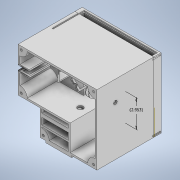
# Autodesk Inventor part: Box
Saved by Autodesk Inventor 2022 (Build 260153000, 153)
## iProperties
Created: 2022-06-14
Part Number: Box
Material: Generic
Document SubType Name: Modeling
Designer: yashm
Density: 1 g/cm^3
Appearance: Default
Author: yashm
Autodesk Inventor part; units mm, degrees
(part 1 of 2)
sketch "Sketch1" plane through (0, 0, 0) normal (0, 0, 1) x (1, 0, 0)
  line L0 (0, 0) -> (145, 0)
  line L1 (145, 0) -> (145, 180)
  line L2 (145, 180) -> (0, 180)
  line L3 (0, 180) -> (0, 0)
  dimension "d0" = 180
  dimension "d1" = 145
  constraints: 8 end point, 2 parallel, 1 horizontal, 1 perpendicular
  measures "d0" distance of L2.end L0.start
  measures "d1" distance of L0.start L0.end
extrude "Extrusion1" add sketch "Sketch1" along normal blind 150
shell "Shell2" thickness 5 outward yes removed faces 1 at (48.3333, 120, 150)
ref_plane "Work Plane1" through (0, 30, 0) normal (0, 1, 0) x (1, 0, 0)
sketch "Sketch4" plane through (0, 30, 0) normal (0, 1, 0) x (1, 0, 0)
  line L0 (53, -95.6365) -> (53, 0)
  line L1 (53, 0) -> (57, 0)
  line L2 (57, 0) -> (57, -95.6365)
  line L3 (0, 0) -> (145, 0) projected
  arc A0 (53, -95.6365) -> (57, -95.6365) centre (55, -100) ccw
  point P0 (55, 0)
  dimension "d8" = 4
  dimension "d10" = 55
  dimension "d12" = 4.8
  dimension "d13" = 100
  constraints: 6 end point, 2 perpendicular, 2 point on circle, 1 centre point, 1 collinear, 1 midpoint, 1 parallel, 1 point on line, 1 vertical
  measures "d8" distance of L0.end L1.end
  measures "d10" distance of L3.start point (55, 0)
  measures "d12" radius of A0
  measures "d13" distance of point (55, 0) A0.centre
extrude "Extrusion2" add sketch "Sketch4" along normal mid plane 4
sketch "Sketch6" plane through (0, 32, 0) normal (0, 1, 0) x (1, 0, 0)
  circle A0 centre (55, -100) radius 2.3
  arc A1 (53, -95.6365) -> (57, -95.6365) centre (55, -100) ccw projected
  point P0 (0, 0)
  dimension "d16" = 4.6
  constraints: 1 centre point, 1 concentric
  measures "d16" diameter of A0
extrude "Extrusion3" cut sketch "Sketch6" against normal blind 4 draft -5
sketch "Sketch8" plane through (0, 30, 0) normal (0, 1, 0) x (1, 0, 0)
  circle A0 centre (55, -100) radius 2.8
  arc A1 (53, -95.6365) -> (57, -95.6365) centre (55, -100) ccw projected
  point P0 (0, 0)
  dimension "d20" = 5.6
  constraints: 1 centre point, 1 concentric
  measures "d20" diameter of A0
extrude "Extrusion4" cut sketch "Sketch8" along normal mid plane 1.3
ref_plane "Work Plane2" through (0, 180, 100) normal (0, 0, 1) x (1, 0, 0)
sketch "Sketch9" plane through (0, 180, 100) normal (0, 0, 1) x (1, 0, 0)
  line L0 (50.2, -152) -> (50.2, -148) projected
  line L1 (59.8, -152) -> (59.8, -148) projected
  line L2 (59.8, -150.6) -> (50.2, -150.6)
  line L3 (50.2, -150.6) -> (50.2, -149.4)
  line L4 (50.2, -149.4) -> (59.8, -149.4)
  line L5 (59.8, -149.4) -> (59.8, -150.6)
  line L6 (59.8, -148) -> (50.2, -148) projected
  point P0 (0, -180)
  point P1 (53, -148)
  point P2 (57, -148)
  point P3 (50.2, -150)
  dimension "d24" = 1.2
  constraints: 8 end point, 3 parallel, 2 midpoint, 1 horizontal, 1 perpendicular
  measures "d24" distance of L2.end L3.end
extrude "Extrusion5" cut sketch "Sketch9" along normal blind 4.8 contours L0 L4 L1 L2
sketch "Sketch10" plane through (0, 180, 100) normal (0, 0, 1) x (1, 0, 0)
  line L0 (52.7, -148) -> (57.3, -148)
  line L1 (57.3, -148) -> (57.3, -152)
  line L2 (57.3, -152) -> (52.7, -152)
  line L3 (52.7, -152) -> (52.7, -148)
  line L4 (52.7, -148) -> (57.3, -148) projected
  line L5 (53, -148) -> (57, -148) projected
  line L6 (53, -148) -> (57, -148) projected
  line L7 (50.2, -152) -> (59.8, -152) projected
  line L8 (52.7, -148) -> (57.3, -148) projected
  line L9 (57, -148) -> (57, -152) projected
  line L10 (57, -148) -> (57, -152) projected
  point P0 (0, -180)
  point P1 (53, -152)
  point P2 (55, -148)
  point P3 (55, -148)
  constraints: 8 end point, 4 midpoint, 2 equal length, 2 parallel, 1 horizontal, 1 perpendicular
extrude "Extrusion6" cut sketch "Sketch10" along normal blind 4.8 contours L0 L9 L2 L3
ref_plane "Work Plane3" through (0, 130, 0) normal (0, 1, 0) x (1, 0, 0)
sketch "Sketch11" plane through (0, 130, 0) normal (0, 1, 0) x (1, 0, 0)
  arc A0 (57, -104.3635) -> (57, -95.6365) centre (55, -100) ccw projected
  line L0 (57, 0) -> (57, -95.6365) projected
  line L1 (53, -95.6365) -> (53, 0) projected
  arc A1 (56.95, -100) -> (53.05, -100) centre (55, -100) ccw projected
  arc A2 (53, -95.6365) -> (52.7, -104.2131) centre (55, -100) ccw projected
  line L2 (52.7, -100) -> (52.7, -104.2131) projected
  line L3 (57, -104.3635) -> (57, -100) projected
  point P0 (0, 0)
sketch "Sketch12" plane through (0, 180, 0) normal (0, 0, 1) x (1, 0, 0)
  line L0 (42.9792, -41.5147) -> (46.5147, -37.9792)
  line L1 (46.5147, -37.9792) -> (67.0208, -58.4853)
  line L2 (67.0208, -58.4853) -> (63.4853, -62.0208)
  line L3 (63.4853, -62.0208) -> (42.9792, -41.5147)
  line L4 (-96, -50) -> (191, -50) projected
  point P0 (0, -180)
  point P1 (55, -50)
  dimension "d30" = 135
  dimension "d31" = 5
  dimension "d32" = 29
  dimension "d33" = 14.5
  dimension "d34" = 2.5
  constraints: 8 end point, 3 perpendicular
  measures "d30" angle of L4 L1
  measures "d31" distance between parallel lines of L1 L3
  measures "d32" distance between parallel lines of L0 L2
  measures "d33" distance from line of point (55, -50) L2
  measures "d34" distance from line of point (55, -50) L3
extrude "Extrusion7" add sketch "Sketch12" along normal blind 115
sketch "Sketch13" plane through (0, 180, 115) normal (0, 0, 1) x (1, 0, 0)
  line L0 (46.5147, -40.8076) -> (64.1924, -58.4853)
  line L1 (64.1924, -58.4853) -> (63.4853, -59.1924)
  line L2 (63.4853, -59.1924) -> (45.8076, -41.5147)
  line L3 (46.5147, -40.8076) -> (45.8076, -41.5147)
  line L4 (63.4853, -62.0208) -> (67.0208, -58.4853) projected
  line L5 (42.9792, -41.5147) -> (63.4853, -62.0208) projected
  line L6 (67.0208, -58.4853) -> (46.5147, -37.9792) projected
  point P0 (0, -180)
  dimension "d41" = 2
  dimension "d42" = 2
  dimension "d43" = 2
  dimension "d44" = 25
  constraints: 8 end point, 2 parallel, 1 perpendicular
  measures "d41" distance between parallel lines of L4 L1
  measures "d42" distance between parallel lines of L5 L2
  measures "d43" distance between parallel lines of L6 L0
  measures "d44" distance between parallel lines of L1 L3
extrude "Extrusion8" cut sketch "Sketch13" against normal blind 27.5
sketch "Sketch14" plane through (63.4853, 117.9792, 115) normal (-0.7071068, -0.7071068, 0) x (-0.7071068, 0.7071068, 0)
  line L0 (95.8173, 120) -> (-38.533, 120) projected
  ellipse E0 centre (14.5, 15) end of major axis (14.5, 10.2) minor radius 3.3941 (16.1263, 10.7869) -> (15.9142, 19.3635) ccw projected
  line L1 (25, 4.5) -> (4, 4.5)
  line L2 (4, 4.5) -> (4, 25.5)
  line L3 (4, 25.5) -> (25, 25.5)
  line L4 (25, 25.5) -> (25, 4.5)
  line L5 (25, 4.5) -> (4, 25.5) construction
  line L6 (4, 4.5) -> (25, 25.5) construction
  point P0 (-38.533, 115)
  dimension "d47" = 21
  dimension "d48" = 21
  constraints: 12 end point, 2 midpoint, 2 parallel, 1 horizontal, 1 perpendicular, 1 other
  measures "d47" distance of L2.end L3.end
  measures "d48" distance of L1.end L2.end
extrude "Extrusion9" cut sketch "Sketch14" against normal blind 5
ref_plane "Work Plane5" through (90, 0, 0) normal (1, 0, 0) x (0, 0, -1)
sketch "Sketch16" plane through (90, 0, 0) normal (1, 0, 0) x (0, 0, -1)
  line L0 (-100, 146.7) -> (0, 146.7)
  line L1 (0, 146.7) -> (0, 113.3)
  line L2 (0, 113.3) -> (-100, 113.3)
  line L3 (-150, 180) -> (-150, 0) projected
  line L4 (0, 121.5147) -> (0, 117.9792) projected
  line L5 (0, 117.9792) -> (0, 138.4853) projected
  line L6 (0, 138.4853) -> (0, 142.0208) projected
  line L7 (0, 142.0208) -> (0, 121.5147) projected
  line L8 (0, 28) -> (0, 32) projected
  line L9 (0, 32) -> (0, 28) projected
  line L10 (0, 0) -> (0, 180) projected
  line L11 (0, 180) -> (0, 0) projected
  arc A0 (-100, 146.7) -> (-100, 113.3) centre (-100, 130) ccw
  point P0 (-100, 130)
  dimension "d370" = 33.4
  dimension "d371" = 0
  dimension "d372" = 16.7
  dimension "d373" = 100
  dimension "d374" = 130
  constraints: 6 end point, 2 point on circle, 1 centre point, 1 point on line
  measures "d370" distance between parallel lines of L2 L0
  measures "d371" horizontal distance of L0.start A0.centre
  measures "d372" radius of A0
  measures "d373" distance from line of L7 A0.centre
  measures "d374" vertical distance of point (0, 0) A0.centre
extrude "Extrusion10" add sketch "Sketch16" along normal mid plane 10
sketch "Sketch17" plane through (95, 0, 0) normal (1, 0, 0) x (0, 0, -1)
  circle A0 centre (-100, 130) radius 10
  arc A1 (-100, 146.7) -> (-100, 113.3) centre (-100, 130) ccw projected
  point P0 (0, 0)
  dimension "d57" = 20
  constraints: 1 centre point, 1 concentric
  measures "d57" diameter of A0
extrude "Extrusion11" cut sketch "Sketch17" against normal blind 14
ref_plane "Work Plane6" through (115, 0, 0) normal (1, 0, 0) x (0, 0, -1)
ref_plane "Work Plane7" through (5, 0, 0) normal (1, 0, 0) x (0, 0, -1)
ref_plane "Work Plane8" through (0, 180, 100) normal (0, 0, 1) x (1, 0, 0)
ref_plane "Work Plane9" through (1460.5, 0, 0) normal (1, 0, 0) x (0, 0, -1)
ref_plane "Work Plane10" through (57.5, 0, 0) normal (1, 0, 0) x (0, 0, -1)
sketch "Sketch27" plane through (0, 0, -5) normal (0, 0, -1) x (-1, 0, 0)
  line L0 (65, 185) -> (5, 185)
  line L1 (5, 185) -> (5, 65)
  line L2 (5, 65) -> (65, 65)
  line L3 (65, 65) -> (65, 185)
  line L4 (5, 185) -> (5, -5) projected
  point P0 (0, 0)
  dimension "d92" = 120
  dimension "d93" = 60
  constraints: 8 end point, 2 parallel, 2 point on line, 1 horizontal, 1 perpendicular
  measures "d92" distance of L0.end L1.end
  measures "d93" distance between parallel lines of L3 L1
extrude "Extrusion18" add sketch "Sketch27" against normal blind 155
sketch "Sketch28" plane through (0, 0, 150) normal (0, 0, 1) x (1, 0, 0)
  line L0 (-60, 180) -> (-5, 180)
  line L1 (-5, 180) -> (-5, 70)
  line L2 (-5, 70) -> (-60, 70)
  line L3 (-60, 70) -> (-60, 180)
  line L4 (-5, 65) -> (-5, -5) projected
  line L5 (-65, 65) -> (-5, 65) projected
  line L6 (-65, 185) -> (-65, 65) projected
  line L7 (150, 185) -> (-65, 185) projected
  point P0 (0, 0)
  point P1 (-5, 185)
  dimension "d96" = 0
  dimension "d97" = 5
  dimension "d98" = 5
  dimension "d99" = 5
  constraints: 8 end point, 2 parallel, 1 horizontal, 1 perpendicular
  measures "d96" distance from line of L4 L1.end
  measures "d97" distance between parallel lines of L5 L2
  measures "d98" distance between parallel lines of L6 L3
  measures "d99" distance between parallel lines of L7 L0
extrude "Extrusion19" cut sketch "Sketch28" against normal blind 200
sketch "Sketch45" plane through (0, 0, -5) normal (0, 0, -1) x (-1, 0, 0)
  line L0 (5, 180) -> (60, 180)
  line L1 (60, 180) -> (60, 70)
  line L2 (60, 70) -> (5, 70)
  line L3 (5, 70) -> (5, 180)
  point P0 (0, 0)
  constraints: 8 end point, 3 coincident, 2 parallel, 1 horizontal, 1 perpendicular
extrude "Extrusion29" add sketch "Sketch45" against normal blind 5
sketch "Sketch57" plane through (0, 0, 150) normal (0, 0, 1) x (1, 0, 0)
  line L0 (145, 180) -> (0, 180) projected
  line L1 (-5, 70) -> (-60, 70) projected
  line L2 (0, 180) -> (-5, 180)
  line L3 (-5, 180) -> (-5, 70)
  line L4 (-5, 70) -> (0, 70)
  line L5 (0, 70) -> (0, 180)
  point P0 (0, 0)
  constraints: 8 end point, 2 parallel, 1 horizontal, 1 perpendicular
extrude "Extrusion36" cut sketch "Sketch57" against normal blind 150
ref_plane "Work Plane12" through (115, 0, 150) normal (1, 0, 0) x (0, 0, -1)
sketch "Sketch64" plane through (-60, 70, 150) normal (1, 0, 0) x (0, 0, -1)
  line L0 (62, 66) -> (0, 66)
  line L1 (0, 66) -> (0, 70)
  line L2 (0, 70) -> (66, 70)
  line L3 (66, 70) -> (66, 50)
  line L4 (66, 50) -> (0, 50)
  line L5 (0, 50) -> (0, 54)
  line L6 (0, 54) -> (62, 54)
  line L7 (62, 54) -> (62, 66)
  circle A0 centre (50, 60) radius 10 projected
  line L8 (0, 0) -> (0, 110) projected
  point P0 (150, -70)
  point P1 (0, 68)
  dimension "d219" = 4
  dimension "d220" = 4
  dimension "d221" = 12
  dimension "d223" = 6
  dimension "d224" = 12
  constraints: 16 end point, 6 perpendicular, 2 equal length, 1 horizontal, 1 midpoint, 1 parallel, 1 point on line
  measures "d219" distance of L0.end L1.end
  measures "d220" distance between parallel lines of L3 L7
  measures "d221" distance of L6.end L0.start
  measures "d223" distance from line of L0 A0.centre
  measures "d224" distance from line of A0.centre L7
extrude "Extrusion43" add sketch "Sketch64" along normal blind 25 contours L0 A0 L2 L3 L4 L6 L7 | L0 A0 | L0 L1 L2 A0 | A0 L6 | A0 L4 L5 L6
sketch "Sketch67" plane through (-65, 65, -5) normal (-1, 0, 0) x (0, 0, 1)
  line L0 (89, 75) -> (155, 75) projected
  line L1 (89, 55) -> (89, 75) projected
  line L2 (155, 55) -> (89, 55) projected
  line L3 (89, 55) -> (155, 55) projected
  line L4 (89, 55) -> (89, 75)
  line L5 (155, 75) -> (89, 75) projected
  line L6 (89, 75) -> (155, 75)
  line L7 (155, 75) -> (155, 55)
  line L8 (155, 55) -> (89, 55)
  line L9 (155, 120) -> (155, 0) projected
  point P0 (5, -65)
  point P1 (155, 65)
  point P2 (118, 75)
  constraints: 8 end point, 2 perpendicular, 2 point on line, 1 collinear, 1 midpoint
extrude "Extrusion44" cut sketch "Sketch67" against normal blind 3
sketch "Sketch68" plane through (-62, 65, -5) normal (-1, 0, 0) x (0, 0, 1)
  line L0 (155, 71) -> (93, 71) projected
  line L1 (93, 71) -> (93, 59) projected
  line L2 (89, 55) -> (89, 75) projected
  line L3 (89, 75) -> (155, 75) projected
  line L4 (93, 59) -> (155, 59) projected
  line L5 (155, 55) -> (89, 55) projected
  line L6 (91, 73) -> (91, 57)
  line L7 (91, 57) -> (155, 57)
  line L8 (155, 57) -> (155, 73)
  line L9 (155, 73) -> (91, 73)
  line L10 (155, 75) -> (155, 55) projected
  point P0 (5, -65)
  dimension "d229" = 2
  dimension "d230" = 2
  dimension "d231" = 2
  dimension "d232" = 0
  constraints: 8 end point, 3 perpendicular, 1 vertical
  measures "d229" distance between parallel lines of L9 L0
  measures "d230" distance between parallel lines of L6 L1
  measures "d231" distance between parallel lines of L7 L4
  measures "d232" distance between parallel lines of L8 L10
extrude "Extrusion45" cut sketch "Sketch68" against normal blind 2 contours L8 L4 L1 L0 | L0 L1 L4 L8 L7 L6 L9
ref_plane "Work Plane13" through (0, 0, 65) normal (0, 0, 1) x (1, 0, 0)
sketch "Sketch71" plane through (0, 0, 65) normal (0, 0, 1) x (1, 0, 0)
  line L0 (145, 180) -> (-60, 180) projected
  line L1 (-60, 180) -> (30, 180)
  line L2 (30, 180) -> (30, 70)
  line L3 (30, 70) -> (-60, 70)
  line L4 (-60, 70) -> (-60, 180)
  line L5 (0, 70) -> (-60, 70) projected
  point P0 (0, 0)
  point P1 (30, 180)
  dimension "d236" = 90
  constraints: 8 end point, 2 parallel, 1 horizontal, 1 perpendicular, 1 point on line
  measures "d236" distance between parallel lines of L4 L2
extrude "Extrusion46" add sketch "Sketch71" along normal mid plane 4
sketch "Sketch74" plane through (0, 0, 67) normal (0, 0, 1) x (1, 0, 0)
  line L0 (0, 70) -> (30, 70) projected
  line L1 (0, 70) -> (30, 70)
  line L2 (30, 70) -> (30, 180) projected
  line L3 (30, 70) -> (30, 180)
  line L4 (30, 180) -> (27, 180)
  line L5 (-60, 180) -> (30, 180) projected
  line L6 (30, 180) -> (27, 180)
  line L7 (27, 180) -> (27, 73)
  line L8 (27, 73) -> (0, 73)
  line L9 (0, 73) -> (0, 70)
  point P0 (0, 0)
  dimension "d239" = 3
  dimension "d240" = 3
  constraints: 14 end point, 3 collinear, 2 perpendicular, 1 point on line, 1 vertical
  measures "d239" distance between parallel lines of L8 L0
  measures "d240" distance between parallel lines of L2 L7
extrude "Extrusion47" add sketch "Sketch74" against normal through all
sketch "Sketch76" plane through (-65, 65, -5) normal (-1, 0, 0) x (0, 0, 1)
  line L0 (68.001, 120) -> (68.001, 0)
  line L1 (68, 115) -> (68, 5) projected
  line L2 (155, 0) -> (0, 0) projected
  line L3 (68.001, 0) -> (0, 0)
  line L4 (0, 0) -> (0, 120) projected
  line L5 (0, 0) -> (0, 120)
  line L6 (0, 120) -> (68.001, 120)
  line L7 (0, 120) -> (155, 120) projected
  point P0 (5, -65)
  point P1 (68.001, 0)
  constraints: 6 end point, 3 collinear, 1 vertical, 3 other
extrude "Extrusion48" cut sketch "Sketch76" against normal blind 5
ref_plane "Work Plane14" through (-25, 70, 150) normal (1, 0, 0) x (0, 0, -1)
sketch "Sketch85" plane through (0, 0, 67) normal (0, 0, 1) x (1, 0, 0)
  line L0 (-32.5, 136) -> (-20.5, 136)
  line L1 (-20.5, 136) -> (-20.5, 124)
  line L2 (-20.5, 124) -> (-32.5, 124)
  line L3 (-32.5, 124) -> (-32.5, 136)
  line L4 (-60, 124) -> (-35, 124) projected
  line L5 (-60, 136) -> (-35, 136) projected
  line L6 (-60, 124) -> (-60, 136) projected
  line L7 (-35, 136) -> (-35, 124) projected
  point P0 (0, 0)
  dimension "d275" = 12
  dimension "d571" = 12
  dimension "d572" = 25
  dimension "d575" = 0
  constraints: 8 end point, 2 parallel, 2 perpendicular, 1 horizontal
  measures "d275" distance of L0.start L0.end
  measures "d571" distance between parallel lines of L4 L5
  measures "d572" distance between parallel lines of L6 L7
  measures "d575" distance between parallel lines of L5 L0
extrude "sample lens stand" add sketch "Sketch85" along normal blind 19.74 contours L0 L1 L2 L3
ref_plane "Work Plane15" through (0, 0, 77) normal (0, 0, 1) x (1, 0, 0)
ref_plane "Work Plane21" through (0, 0, 79) normal (0, 0, 1) x (1, 0, 0)
sketch "Sketch89" plane through (0, 0, 67) normal (0, 0, 1) x (1, 0, 0)
  line L0 (-12.14, 140) -> (-8.14, 140)
  line L1 (-8.14, 140) -> (-8.14, 144)
  line L2 (-8.14, 144) -> (-12.14, 144)
  line L3 (-12.14, 144) -> (-12.14, 140)
  circle A0 centre (-5.14, 130) radius 5 projected
  line L4 (-35, 140) -> (-35, 136) projected
  point P0 (0, 0)
  dimension "d285" = 4
  dimension "d286" = 4
  dimension "d287" = 10
  dimension "d309" = 3
  dimension "d682" = 22.86
  constraints: 8 end point, 2 parallel, 1 horizontal, 1 perpendicular
  measures "d285" distance of L2.end L0.start
  measures "d286" distance of L1.end L2.end
  measures "d287" distance from line of L0 A0.centre
  measures "d309" distance from line of A0.centre L1
  measures "d682" distance between parallel lines of L4 L3
extrude "Extrusion57" add sketch "Sketch89" along normal blind 35 contours L3 L2 L1 L0
sketch "Sketch90" plane through (-12.14, 140, 67) normal (0, -1, 0) x (1, 0, 0)
  line L0 (-2.7175, 26.1109) -> (14.9602, 43.7886)
  line L1 (14.9602, 43.7886) -> (17.7886, 40.9602)
  line L2 (17.7886, 40.9602) -> (0.1109, 23.2825)
  line L3 (0.1109, 23.2825) -> (-2.7175, 26.1109)
  line L4 (0, 0) -> (0, 35) projected
  line L5 (0, 35) -> (4, 35) projected
  point P0 (12.14, -67)
  point P1 (4, 30)
  dimension "d291" = 45
  dimension "d292" = 5
  dimension "d293" = 4
  dimension "d294" = 25
  dimension "d295" = 2
  dimension "d296" = 7.5
  dimension "d297" = 4
  constraints: 8 end point, 3 perpendicular
  measures "d291" angle of L4 L0
  measures "d292" distance from line of point (4, 30) L5
  measures "d293" distance between parallel lines of L2 L0
  measures "d294" distance between parallel lines of L1 L3
  measures "d295" distance from line of L2 point (4, 30)
  measures "d296" distance from line of L3 point (4, 30)
  measures "d297" distance from line of L4 point (4, 30)
extrude "Extrusion58" add sketch "Sketch90" along normal blind 30 and the other way blind 30
sketch "Sketch91" plane through (-14.8575, 110, 93.1109) normal (-0.7071068, 0, 0.7071068) x (0.7071068, 0, 0.7071068)
  line L0 (3, 60) -> (22, 60)
  line L1 (22, 60) -> (22, 3)
  line L2 (22, 3) -> (3, 3)
  line L3 (3, 3) -> (3, 60)
  line L4 (0, 60) -> (25, 60) projected
  line L5 (25, 0) -> (0, 0) projected
  line L6 (25, 60) -> (25, 0) projected
  line L7 (0, 60) -> (0, 0) projected
  point P0 (-55.3335, -110)
  dimension "d302" = 3
  dimension "d303" = 3
  dimension "d304" = 3
  constraints: 8 end point, 2 parallel, 1 horizontal, 1 perpendicular, 1 point on line
  measures "d302" distance between parallel lines of L5 L2
  measures "d303" distance between parallel lines of L6 L1
  measures "d304" distance between parallel lines of L7 L3
extrude "Extrusion59" cut sketch "Sketch91" along normal blind 5 and the other way blind 10 contours L0 L1 L2 L3
sketch "Sketch94" plane through (-12.14, 170, 67) normal (0, 1, 0) x (1, 0, 0)
  line L0 (14.9602, -41.6673) -> (-0.5962, -26.1109)
  line L1 (-0.5962, -26.1109) -> (0.1109, -25.4038)
  line L2 (0.1109, -25.4038) -> (15.6673, -40.9602)
  line L3 (15.6673, -40.9602) -> (14.9602, -41.6673)
  line L4 (-2.7175, -26.1109) -> (-0.5962, -28.2322) projected
  line L5 (0.1109, -23.2825) -> (-2.7175, -26.1109) projected
  line L6 (14.9602, -43.7886) -> (17.7886, -40.9602) projected
  line L7 (2.2322, -25.4038) -> (0.1109, -23.2825) projected
  line L8 (12.8388, -41.6673) -> (14.9602, -43.7886) projected
  point P0 (12.14, 67)
  dimension "d310" = 25
  dimension "d311" = 4
  dimension "d312" = 1.5
  dimension "d313" = 1.5
  dimension "d314" = 1.5
  dimension "d315" = 1.5
  constraints: 8 end point, 4 parallel
  measures "d310" distance between parallel lines of L6 L5
  measures "d311" distance between parallel lines of L7 L4
  measures "d312" distance between parallel lines of L5 L1
  measures "d313" distance between parallel lines of L6 L3
  measures "d314" distance between parallel lines of L8 L0
  measures "d315" distance between parallel lines of L7 L2
extrude "Extrusion60" cut sketch "Sketch94" against normal blind 42
sketch "Sketch98" plane through (0, 0, 0) normal (0, 0, 1) x (1, 0, 0)
  line L0 (0, 65) -> (0, 70)
  line L1 (0, 70) -> (77, 70)
  line L2 (77, 70) -> (77, 0)
  line L3 (77, 0) -> (72, 0)
  line L4 (72, 0) -> (72, 65)
  line L5 (72, 65) -> (0, 65)
  line L6 (-65, 65) -> (-5, 65) projected
  line L7 (0, 70) -> (-60, 70) projected
  line L8 (145, 0) -> (0, 0) projected
  line L9 (57, 32) -> (57, 28) projected
  point P0 (74.5, 0)
  dimension "d328" = 5
  dimension "d329" = 5
  dimension "d330" = 15
  constraints: 12 end point, 6 perpendicular, 1 midpoint, 1 point on line, 1 vertical
  measures "d328" distance of L2.end L3.end
  measures "d329" distance between parallel lines of L6 L7
  measures "d330" distance between parallel lines of L9 L4
extrude "Extrusion64" add sketch "Sketch98" along normal blind 150
sketch "Sketch99" plane through (-60, 70, 67) normal (0, 1, 0) x (1, 0, 0)
  circle A0 centre (115, -33) radius 7.5
  arc A1 (117, -37.3635) -> (117, -28.6365) centre (115, -33) ccw projected
  point P0 (60, 67)
  dimension "d333" = 15
  constraints: 1 centre point, 1 concentric
  measures "d333" diameter of A0
extrude "Extrusion65" cut sketch "Sketch99" against normal blind 5
ref_plane "Work Plane16" through (0, 0, -20) normal (0, 0, -1) x (-1, 0, 0)
sketch "Sketch111" plane through (63.4853, 117.9792, 115) normal (-0.7071068, -0.7071068, 0) x (-0.7071068, 0.7071068, 0)
  line L0 (0, 115) -> (0, 0) projected
  line L1 (29, 115) -> (29, 0) projected
  arc A0 (18.5, 0) -> (10.5, 0) centre (14.5, 0) ccw
  line L2 (29, 0) -> (0, 0) projected
  line L3 (18.5, 0) -> (10.5, 0)
  line L4 (4, 4.5) -> (25, 4.5) projected
  point P0 (-38.533, 115)
  dimension "d382" = 29
  dimension "d383" = 14.5
  dimension "d384" = 4
  constraints: 2 end point, 2 point on circle, 1 centre point, 1 midpoint, 1 parallel, 1 point on line
  measures "d382" distance between parallel lines of L0 L1
  measures "d383" distance from line of L1 A0.centre
  measures "d384" radius of A0
extrude "Extrusion69" cut sketch "Sketch111" against normal blind 5
sketch "Sketch112" plane through (150, -5, -5) normal (1, 0, 0) x (0, 0, -1)
  circle A0 centre (-105, 135) radius 10 projected
  circle A1 centre (-105, 135) radius 5
  point P0 (-5, 5)
  dimension "d387" = 10
  constraints: 1 centre point, 1 coincident
  measures "d387" diameter of A1
extrude "Extrusion70" cut sketch "Sketch112" against normal blind 5 contours A1
sketch "Sketch114" plane through (0, 0, -5) normal (0, 0, -1) x (-1, 0, 0)
  line L0 (5, -5) -> (-150, -5) projected
  line L1 (5, -5) -> (-150, -5)
  line L2 (-150, -5) -> (-150, 185) projected
  line L3 (-150, -5) -> (-150, 185)
  line L4 (-150, 185) -> (60, 185) projected
  line L5 (-150, 185) -> (60, 185)
  line L6 (5, 65) -> (60, 65) projected
  line L7 (60, 185) -> (60, 65)
  line L8 (5, 65) -> (5, -5) projected
  line L9 (60, 65) -> (5, 65)
  line L10 (5, 65) -> (5, -5)
  point P0 (0, 0)
  constraints: 12 end point, 3 collinear, 2 perpendicular, 1 horizontal
extrude "Extrusion71" add sketch "Sketch114" along normal blind 20
sketch "Sketch115" plane through (-5, -5, 150) normal (0, -1, 0) x (1, 0, 0)
  line L0 (150, -170) -> (5, -170)
  line L1 (5, -170) -> (5, -155)
  line L2 (5, -155) -> (150, -155)
  line L3 (150, -155) -> (150, -170)
  line L4 (155, -175) -> (0, -175) projected
  line L5 (155, 0) -> (155, -175) projected
  line L6 (0, -175) -> (0, 0) projected
  point P0 (5, -150)
  dimension "d393" = 5
  dimension "d394" = 5
  dimension "d395" = 5
  dimension "d396" = 15
  constraints: 8 end point, 2 parallel, 1 horizontal, 1 perpendicular
  measures "d393" distance between parallel lines of L0 L4
  measures "d394" distance between parallel lines of L3 L5
  measures "d395" distance between parallel lines of L6 L1
  measures "d396" distance between parallel lines of L0 L2
extrude "Extrusion72" cut sketch "Sketch115" against normal blind 67
sketch "Sketch117" plane through (-65, 185, 150) normal (0, 1, 0) x (1, 0, 0)
  line L0 (10, 170) -> (210, 170)
  line L1 (210, 170) -> (210, 155)
  line L2 (210, 155) -> (10, 155)
  line L3 (10, 155) -> (10, 170)
  line L4 (5, 86.999) -> (5, 175) projected
  line L5 (215, 175) -> (215, 0) projected
  line L6 (5, 175) -> (215, 175) projected
  point P0 (65, 150)
  dimension "d401" = 15
  dimension "d402" = 5
  dimension "d403" = 5
  dimension "d404" = 5
  constraints: 8 end point, 2 parallel, 1 horizontal, 1 perpendicular
  measures "d401" distance of L0.end L1.end
  measures "d402" distance between parallel lines of L4 L3
  measures "d403" distance between parallel lines of L5 L1
  measures "d404" distance between parallel lines of L0 L6
extrude "Extrusion73" cut sketch "Sketch117" against normal blind 117
sketch "Sketch124" plane through (-5, -5, 150) normal (0, -1, 0) x (1, 0, 0)
  arc A0 (57.8181, -50) -> (62, -49.1279) centre (60, -50) ccw projected
  circle A1 centre (60, -50) radius 5
  point P0 (5, -150)
  constraints: 1 centre point, 1 coincident
extrude "Extrusion78" cut sketch "Sketch124" against normal blind 10
sketch "Sketch125" plane through (0, 0, 150) normal (0, 1, 0) x (1, 0, 0)
  circle A0 centre (55, 50) radius 5 projected
  circle A1 centre (55, 50) radius 5
  point P0 (0, 150)
  constraints: 1 centre point, 1 coincident
extrude "Extrusion79" add sketch "Sketch125" along normal mid plane 2.6
sketch "Sketch126" plane through (55, 1.3, 100) normal (0, 1, 0) x (1, 0, 0)
  circle A0 centre (0, 0) radius 1.775
  point P0 (-55, 100)
  dimension "d423" = 3.55
  constraints: 1 centre point
  measures "d423" diameter of A0
extrude "Extrusion80" cut sketch "Sketch126" against normal blind 2.6
sketch "Sketch127" plane through (55, -1.3, 100) normal (0, -1, 0) x (1, 0, 0)
  circle A0 centre (0, 0) radius 2.8
  point P0 (-55, -100)
  dimension "d426" = 5.6
  constraints: 1 centre point
  measures "d426" diameter of A0
extrude "Extrusion81" cut sketch "Sketch127" against normal blind 1.2
sketch "Sketch128" plane through (55, -0.1, 100) normal (0, -1, 0) x (1, 0, 0)
  circle A0 centre (0, 0) radius 2.1
  point P0 (-55, -100)
  dimension "d429" = 4.2
  constraints: 1 centre point
  measures "d429" diameter of A0
extrude "Extrusion82" cut sketch "Sketch128" against normal blind 0.1
sketch "Sketch131" plane through (0, 0, 67) normal (0, 0, 1) x (1, 0, 0)
  line L0 (-9.9078, 170) -> (-9.9078, 144) projected
  line L1 (-14.8575, 170) -> (-12.7362, 170) projected
  line L2 (5.6486, 170) -> (5.6486, 110) construction
  line L3 (2.8202, 110) -> (-14.8575, 110) projected
  line L4 (5.6486, 110) -> (2.8202, 110) projected
  line L5 (-14.8575, 110) -> (5.6486, 110)
  line L6 (0.6988, 170) -> (5.6486, 170)
  line L7 (5.6486, 161.5372) -> (5.6486, 170)
  line L8 (-60, 70) -> (-60, 180) projected
  line L9 (-14.8575, 170) -> (-9.9078, 170)
  line L10 (-9.9078, 113) -> (0.6988, 113)
  line L11 (-14.8575, 170) -> (-14.8575, 110) projected
  line L12 (-9.9078, 170) -> (-9.9078, 144)
  line L13 (-60, 65) -> (-60, 185) projected
  line L14 (-9.9078, 144) -> (-14.8575, 144)
  line L15 (-14.8575, 170) -> (-14.8575, 144)
  line L16 (-14.8575, 110) -> (-14.8575, 113)
  line L17 (0.6988, 113) -> (-14.8575, 113)
  line L18 (-35, 124) -> (-35, 120) projected
  line L19 (0.6988, 170) -> (0.6988, 140)
  line L20 (0.6988, 140) -> (5.6486, 140)
  line L21 (5.6486, 161.5372) -> (5.6486, 140)
  line L22 (0.6988, 113) -> (5.6486, 113)
  line L23 (5.6486, 110) -> (5.6486, 113)
  point P0 (0, 0)
  constraints: 30 end point, 5 perpendicular, 5 point on line, 2 collinear, 1 horizontal, 1 midpoint, 1 parallel, 1 vertical
extrude "Extrusion85" add sketch "Sketch131" along normal up to surface surface through (-12.0291, 140, 90.2825) normal (0.7071068, 0, -0.7071068)
sketch "Sketch132" plane through (-12.14, 170, 67) normal (0, 1, 0) x (1, 0, 0)
  line L0 (14.6066, -39.8995) -> (15.6673, -40.9602) projected
  line L1 (14.6066, -39.8995) -> (14.3102, -37.4818)
  line L2 (15.6673, -38.8388) -> (12.8388, -36.0104) projected
  line L3 (15.6673, -38.8388) -> (14.6066, -39.8995) projected
  line L4 (15.6673, -38.8388) -> (14.6066, -39.8995)
  line L5 (14.3102, -37.4818) -> (15.6673, -38.8388)
  line L6 (-2.7175, -26.1109) -> (-2.7175, -20.4541)
  line L7 (-2.7175, -20.4541) -> (0.1109, -23.2825)
  line L8 (0.1109, -23.2825) -> (-2.7175, -20.4541) projected
  line L9 (0.1109, -23.2825) -> (-2.7175, -26.1109) projected
  line L10 (-2.7175, -26.1109) -> (0.1109, -23.2825)
  point P0 (12.14, 67)
  constraints: 13 end point, 3 collinear, 1 point on line, 1 vertical
extrude "Extrusion86" add sketch "Sketch132" against normal blind 44
sketch "Sketch134" plane through (145, 0, 0) normal (0, 0, 1) x (1, 0, 0)
  line L0 (-68, 70) -> (-205, 70) projected
  line L1 (-150, -5) -> (5, -5) projected
  point P0 (-145, 0)
  dimension "d444" = 75
  measures "d444" distance between parallel lines of L0 L1
sketch "Sketch135" plane through (0, 0, 150) normal (0, 0, 1) x (1, 0, 0)
  line L0 (-60, 160) -> (-60, 179.9274)
  line L1 (-60, 185) -> (-60, 65) projected
  line L2 (27, 180) -> (-60, 180) projected
  line L3 (-60, 180) -> (-40, 180)
  arc A0 (-60, 160) -> (-40, 180) centre (-60, 180) ccw
  line L4 (145, 160) -> (145, 180)
  line L5 (145, 180) -> (125, 180)
  line L6 (145, 20) -> (145, 0)
  line L7 (145, 0) -> (125, 0)
  line L8 (20, 0) -> (0, 0)
  line L9 (0, 0) -> (0, 20)
  line L10 (0, -5) -> (0, 62) projected
  line L11 (-40, 70) -> (-60, 70)
  line L12 (-60, 70) -> (-60, 90)
  arc A1 (125, 180) -> (145, 160) centre (145, 180) ccw
  arc A2 (145, 20) -> (125, 0) centre (145, 0) ccw
  arc A3 (20, 0) -> (0, 20) centre (0, 0) ccw
  arc A4 (-40, 70) -> (-60, 90) centre (-60, 70) ccw
  dimension "d446" = 20
  constraints: 22 end point, 10 point on circle, 7 coincident, 5 centre point, 4 equal radius, 3 perpendicular, 2 horizontal, 2 point on line, 2 vertical, 1 collinear
  measures "d446" distance of L4.start L4.end
extrude "Extrusion87" add sketch "Sketch135" against normal up to next
sketch "Sketch137" plane through (-12.7362, 128, 93.1109) normal (0.7071068, 0, 0.7071068) x (0.7071068, 0, -0.7071068)
  line L0 (1, 0) -> (0, 0)
  line L1 (0, 0) -> (0, 42) projected
  line L2 (1, 0) -> (0, 0)
  line L3 (0, 0) -> (0, 25)
  line L4 (0, 25) -> (1, 25)
  line L5 (1, 25) -> (1, 0)
  point P0 (74.8452, -128)
  point P1 (0, 1)
  dimension "d449" = 25
  constraints: 10 end point, 2 parallel, 1 horizontal, 1 perpendicular, 1 point on line
  measures "d449" distance of L4.end L0.start
sketch "Sketch138" plane through (2.8202, 110, 110.7886) normal (-0.7071068, 0, 0.7071068) x (0.7071068, 0, 0.7071068)
  line L0 (-23.5, 60) -> (-23.5, 18) projected
  line L1 (-1.5, 60) -> (-1.5, 18) projected
  line L2 (-23.5, 60) -> (-1.5, 60)
  line L3 (-1.5, 60) -> (-1.5, 41.5)
  line L4 (-1.5, 41.5) -> (-23.5, 41.5)
  line L5 (-23.5, 41.5) -> (-23.5, 60)
  point P0 (-80.3335, -110)
  point P1 (-23.5, 43)
  point P2 (-23.5, 43)
  point P3 (-23.5, 43)
  dimension "d450" = 1.5
  constraints: 8 end point, 2 parallel, 1 horizontal, 1 perpendicular, 1 point on line
  measures "d450" distance from line of L4 point (-23.5, 43)
extrude "Extrusion88" add sketch "Sketch138" against normal blind 4
extrude "Extrusion89" cut sketch "Sketch137" along normal blind 30
sketch "Sketch139" plane through (0, 0, 150) normal (0, 0, 1) x (1, 0, 0)
  line L0 (72, 0) -> (72, 65) projected
  line L1 (42, 27) -> (72, 27)
  line L2 (72, 27) -> (72, 22)
  line L3 (72, 22) -> (42, 22)
  line L4 (42, 22) -> (42, 27)
  line L5 (72, 0) -> (20, 0) projected
  point P0 (0, 0)
  dimension "d455" = 30
  dimension "d456" = 5
  dimension "d592" = 22
  constraints: 8 end point, 2 parallel, 1 horizontal, 1 perpendicular, 1 point on line
  measures "d455" distance of L2.end L3.end
  measures "d456" distance between parallel lines of L3 L1
  measures "d592" distance between parallel lines of L5 L3
extrude "Extrusion90" add sketch "Sketch139" against normal up to surface (150 mm away)
sketch "Sketch145" plane through (42, 22, 150) normal (0, -1, 0) x (1, 0, 0)
  circle A0 centre (13, -50) radius 5
  circle A1 centre (13, -50) radius 5 projected
  point P0 (-42, -150)
  constraints: 2 concentric, 1 centre point
extrude "Extrusion95" cut sketch "Sketch145" against normal blind 10
sketch "Sketch146" plane through (42, 27, 150) normal (0, 1, 0) x (1, 0, 0)
  circle A0 centre (13, 50) radius 5
  circle A1 centre (13, 50) radius 5 projected
  circle A2 centre (13, 50) radius 5 projected
  point P0 (-42, 150)
  constraints: 2 concentric, 1 centre point
extrude "Extrusion96" add sketch "Sketch146" along normal mid plane 2.6
sketch "Sketch147" plane through (55, 28.3, 100) normal (0, 1, 0) x (1, 0, 0)
  circle A0 centre (0, 0) radius 1.775
  arc A1 (-2, 4.5826) -> (2, 4.5826) centre (0, 0) ccw projected
  circle A2 centre (0, 0) radius 1.775 projected
  point P0 (-55, 100)
  constraints: 2 concentric, 1 centre point
extrude "Extrusion97" cut sketch "Sketch147" against normal blind 2.6
sketch "Sketch148" plane through (55, 25.7, 100) normal (0, -1, 0) x (1, 0, 0)
  circle A0 centre (0, 0) radius 2.8
  circle A1 centre (0, 0) radius 5 projected
  circle A2 centre (0, 0) radius 2.8 projected
  point P0 (-55, -100)
  constraints: 2 concentric, 1 centre point
extrude "Extrusion98" cut sketch "Sketch148" against normal blind 1.2 contours A0
sketch "Sketch150" plane through (55, 26.9, 100) normal (0, -1, 0) x (1, 0, 0)
  circle A0 centre (0, 0) radius 2.1
  point P0 (-55, -100)
  constraints: 1 centre point
extrude "Extrusion99" cut sketch "Sketch150" against normal blind 0.1
sketch "Sketch151" plane through (55, 1.3, 100) normal (0, 1, 0) x (1, 0, 0)
  circle A0 centre (0, 0.3376) radius 2.6209
  point P0 (-55, 100)
  constraints: 1 centre point
extrude "Extrusion100" add sketch "Sketch151" against normal blind 3
ref_plane "Work Plane18" through (90, 0, 0) normal (1, 0, 0) x (0, 0, -1)
sketch "Sketch153" plane through (90, 0, 0) normal (1, 0, 0) x (0, 0, -1)
  circle A0 centre (-100, 130) radius 12.7
  circle A1 centre (-100, 130) radius 10 projected
  point P0 (0, 0)
  dimension "d487" = 25.4
  constraints: 1 centre point, 1 concentric
  measures "d487" diameter of A0
extrude "Extrusion101" cut sketch "Sketch153" along normal mid plane 7
ref_plane "Work Plane19" through (90, 113.3, 100) normal (0, 0, 1) x (1, 0, 0)
sketch "Sketch155" plane through (90, 113.3, 100) normal (0, 0, 1) x (1, 0, 0)
  line L0 (-3.5, 29.4) -> (3.5, 29.4)
  line L1 (3.5, 29.4) -> (3.5, 4)
  line L2 (3.5, 4) -> (-3.5, 4)
  line L3 (-3.5, 4) -> (-3.5, 29.4)
  line L4 (-3.5, 29.4) -> (-3.5, 4) projected
  line L5 (3.5, 4) -> (3.5, 29.4) projected
  point P0 (-90, -113.3)
  constraints: 8 end point, 3 parallel, 1 horizontal, 1 perpendicular
extrude "Extrusion102" cut sketch "Sketch155" along normal blind 17
sketch "Sketch156" plane through (0, 0, 150) normal (0, 0, 1) x (1, 0, 0)
  line L0 (-65, 120) -> (-65, 140) projected
  line L1 (-65, 140) -> (-62, 140)
  line L2 (-62, 140) -> (-62, 137.9748)
  line L3 (-62, 138) -> (-60, 138) projected
  line L4 (-60, 138) -> (-60, 136.0287)
  line L5 (-60, 140) -> (-60, 120) projected
  line L6 (-62, 138) -> (-60, 138)
  line L7 (-60, 124) -> (-35, 124) projected
  line L8 (-60, 136) -> (-60, 124)
  line L9 (-62, 122) -> (-60, 122) projected
  line L10 (-60, 124) -> (-60, 122)
  line L11 (-60, 122) -> (-62, 122)
  line L12 (-62, 122) -> (-62, 120)
  line L13 (-65, 120) -> (-62, 120) projected
  line L14 (-65, 120) -> (-65, 140)
  line L15 (-65, 120) -> (-62, 120)
  line L16 (-62, 120) -> (-62, 122)
  point P0 (0, 0)
  constraints: 22 end point, 2 collinear, 1 horizontal, 1 perpendicular, 1 point on line, 1 vertical
extrude "Extrusion103" add sketch "Sketch156" against normal up to surface (66 mm away)
sketch "Sketch157" plane through (-60, 124, 150) normal (1, 0, 0) x (0, 0, -1)
  line L0 (0, 0) -> (62, 0) projected
  line L1 (0, 12) -> (62, 12)
  line L2 (62, 12) -> (62, 0)
  line L3 (62, 0) -> (0, 0)
  line L4 (0, 0) -> (0, 12)
  point P0 (150, -124)
  constraints: 8 end point, 2 parallel, 1 horizontal, 1 perpendicular
extrude "Extrusion104" cut sketch "Sketch157" against normal blind 25.4
sketch "Sketch159" plane through (0, 0, 150) normal (0, 0, 1) x (1, 0, 0)
  line L0 (-64, 138) -> (-61, 138)
  line L1 (-61, 138) -> (-61, 122)
  line L2 (-61, 122) -> (-64, 122)
  line L3 (-64, 122) -> (-64, 138)
  line L4 (-60, 140) -> (-35, 140) projected
  line L5 (-60, 120) -> (-35, 120) projected
  line L6 (-60, 140) -> (-60, 160) projected
  line L7 (-65, 185) -> (-65, 136) projected
  point P0 (0, 0)
  dimension "d496" = 2
  dimension "d497" = 2
  dimension "d498" = 1
  dimension "d499" = 1
  constraints: 8 end point, 2 parallel, 1 horizontal, 1 perpendicular
  measures "d496" distance between parallel lines of L0 L4
  measures "d497" distance between parallel lines of L2 L5
  measures "d498" distance between parallel lines of L6 L1
  measures "d499" distance between parallel lines of L7 L3
extrude "Extrusion105" cut sketch "Sketch159" against normal blind 65
sketch "Sketch161" plane through (0, 0, 150) normal (0, 0, 1) x (1, 0, 0)
  circle A0 centre (-56, 176) radius 3
  circle A1 centre (141, 176) radius 3
  circle A2 centre (141, 4) radius 3
  circle A3 centre (4, 4) radius 3
  circle A4 centre (-56, 74) radius 3
  line L0 (-61, 138) -> (-61, 136) projected
  line L1 (-61, 136) -> (-35, 136) projected
  line L2 (-35, 140) -> (-35, 136) projected
  line L3 (-60, 140) -> (-35, 140) projected
  line L4 (-60, 140) -> (-60, 160) projected
  arc A5 (-60, 160) -> (-40, 180) centre (-60, 180) ccw projected
  line L5 (-40, 180) -> (125, 180) projected
  arc A6 (125, 180) -> (145, 160) centre (145, 180) ccw projected
  line L6 (145, 160) -> (145, 20) projected
  arc A7 (145, 20) -> (125, 0) centre (145, 0) ccw projected
  line L7 (125, 0) -> (77, 0) projected
  line L8 (77, 0) -> (77, 70) projected
  line L9 (77, 70) -> (-40, 70) projected
  arc A8 (-40, 70) -> (-60, 90) centre (-60, 70) ccw projected
  line L10 (-60, 90) -> (-60, 120) projected
  line L11 (-60, 120) -> (-35, 120) projected
  line L12 (-35, 124) -> (-35, 120) projected
  line L13 (-35, 124) -> (-61, 124) projected
  line L14 (-61, 124) -> (-61, 122) projected
  line L15 (-61, 122) -> (-64, 122) projected
  line L16 (-64, 122) -> (-64, 124) projected
  line L17 (-64, 124) -> (-65, 124) projected
  line L18 (-65, 124) -> (-65, 65) projected
  line L19 (-65, 65) -> (-5, 65) projected
  line L20 (-5, 65) -> (-5, -5) projected
  line L21 (-5, -5) -> (150, -5) projected
  line L22 (150, -5) -> (150, 185) projected
  line L23 (150, 185) -> (-65, 185) projected
  line L24 (-65, 185) -> (-65, 136) projected
  line L25 (-65, 136) -> (-64, 136) projected
  line L26 (-64, 136) -> (-64, 138) projected
  line L27 (-64, 138) -> (-61, 138) projected
  arc A9 (20, 0) -> (0, 20) centre (0, 0) ccw projected
  line L28 (0, 20) -> (0, 65) projected
  line L29 (0, 65) -> (72, 65) projected
  line L30 (72, 65) -> (72, 27) projected
  line L31 (72, 27) -> (42, 27) projected
  line L32 (42, 27) -> (42, 22) projected
  line L33 (42, 22) -> (72, 22) projected
  line L34 (72, 22) -> (72, 0) projected
  line L35 (72, 0) -> (20, 0) projected
  line L36 (-55, 185) -> (-55, 68) projected
  dimension "d503" = 4
  dimension "d504" = 4
  dimension "d505" = 4
  dimension "d506" = 4
  dimension "d507" = 4
  dimension "d508" = 4
  dimension "d509" = 4
  dimension "d510" = 4
  dimension "d511" = 4
  dimension "d512" = 4
  dimension "d513" = 1
  dimension "d514" = 6
  constraints: 5 centre point, 4 equal radius
  measures "d503" horizontal distance of A5.centre A0.centre
  measures "d504" horizontal distance of A5.centre A0.centre
  measures "d505" vertical distance of A5.centre A1.centre
  measures "d506" horizontal distance of A1.centre A6.centre
  measures "d507" horizontal distance of A2.centre A7.centre
  measures "d508" horizontal distance of A7.centre A2.centre
  measures "d509" horizontal distance of point (0, 0) A3.centre
  measures "d510" horizontal distance of point (0, 0) A3.centre
  measures "d511" horizontal distance of A8.centre A4.centre
  measures "d512" horizontal distance of A8.centre A4.centre
  measures "d513" distance from line of L36 A0.centre
  measures "d514" diameter of A4
extrude "Extrusion106" cut sketch "Sketch161" against normal blind 50 contours A0 L36 | L36 A0 | A1 | A2 | A3 | A4 L36 | L36 A4
thread "Thread1" size "1/4-20 UNC" class "2B" standard "ANSI Unified Screw Threads" full length
thread "Thread2" size "1/4-20 UNC" class "2B" standard "ANSI Unified Screw Threads" full length
thread "Thread3" size "1/4-20 UNC" class "2B" standard "ANSI Unified Screw Threads" full length
thread "Thread4" size "1/4-20 UNC" class "2B" standard "ANSI Unified Screw Threads" full length
thread "Thread5" size "1/4-20 UNC" class "2B" standard "ANSI Unified Screw Threads" full length
sketch "Sketch162" plane through (0, 0, 150) normal (0, 0, 1) x (1, 0, 0)
  line L0 (51.818, 132.4749) -> (45.8076, 138.4853) projected
  line L1 (46.5147, 139.1924) -> (52.5251, 133.182) projected
  line L2 (-58, 138) -> (-37, 138)
  line L3 (-37, 138) -> (-37, 137)
  line L4 (-37, 137) -> (-58, 137)
  line L5 (-58, 137) -> (-58, 138)
  line L6 (-35, 140) -> (-35, 136) projected
  line L7 (-60, 140) -> (-60, 160) projected
  line L8 (-61, 136) -> (-35, 136) projected
  line L9 (-58, 123) -> (-37, 123)
  line L10 (-37, 123) -> (-37, 122)
  line L11 (-37, 122) -> (-58, 122)
  line L12 (-58, 122) -> (-58, 123)
  line L13 (-35, 124) -> (-61, 124) projected
  line L14 (-35, 124) -> (-35, 120) projected
  point P0 (0, 0)
  dimension "d527" = 1
  dimension "d528" = 2
  dimension "d529" = 2
  dimension "d530" = 1
  dimension "d531" = 1
  dimension "d532" = 1
  dimension "d533" = 2
  constraints: 16 end point, 4 parallel, 2 equal length, 2 horizontal, 2 perpendicular
  measures "d527" distance between parallel lines of L0 L1
  measures "d528" distance between parallel lines of L6 L3
  measures "d529" distance between parallel lines of L7 L5
  measures "d530" distance of L2.end L3.end
  measures "d531" distance between parallel lines of L8 L4
  measures "d532" distance between parallel lines of L13 L9
  measures "d533" distance between parallel lines of L10 L14
extrude "Extrusion107" cut sketch "Sketch162" against normal blind 66
sketch "Sketch163" plane through (-35, 136, 88) normal (0, -1, 0) x (1, 0, 0)
  line L0 (-21, 2) -> (-4, 2)
  line L1 (-4, 2) -> (-4, 57)
  line L2 (-4, 57) -> (-21, 57)
  line L3 (-21, 57) -> (-21, 2)
  line L4 (-26, 62) -> (0, 62) projected
  line L5 (0, 0) -> (-26, 0) projected
  point P0 (35, -88)
  point P1 (-23, 62)
  point P2 (-2, 62)
  dimension "d536" = 5
  dimension "d537" = 2
  dimension "d538" = 2
  dimension "d539" = 2
  constraints: 8 end point, 2 parallel, 1 horizontal, 1 perpendicular
  measures "d536" distance between parallel lines of L2 L4
  measures "d537" distance between parallel lines of L5 L0
  measures "d538" distance from line of L3 point (-23, 62)
  measures "d539" distance from line of point (-2, 62) L1
extrude "Extrusion108" cut sketch "Sketch163" against normal blind 2
sketch "Sketch164" plane through (-35, 124, 150) normal (0, 1, 0) x (1, 0, 0)
  line L0 (-21, 60) -> (-21, 5) projected
  line L1 (-21, 5) -> (-4, 5) projected
  line L2 (-4, 5) -> (-4, 60) projected
  line L3 (-4, 60) -> (-21, 60) projected
  point P0 (35, 150)
extrude "Extrusion109" cut sketch "Sketch164" against normal blind 2
sketch "Sketch166" plane through (30, 70, 0) normal (0, 0, 1) x (1, 0, 0)
  line L0 (75, 70) -> (95, 70)
  line L1 (95, 70) -> (95, 50)
  line L2 (95, 50) -> (75, 50)
  line L3 (75, 50) -> (75, 70)
  line L4 (115, 90) -> (115, -50) projected
  line L5 (55, 43.3) -> (65, 43.3) projected
  line L6 (65, 76.7) -> (55, 76.7) projected
  point P0 (-30, -70)
  point P1 (75, 60)
  dimension "d547" = 20
  dimension "d548" = 20
  dimension "d549" = 20
  dimension "d550" = 33.4
  dimension "d551" = 16.7
  constraints: 8 end point, 2 parallel, 1 horizontal, 1 midpoint, 1 perpendicular
  measures "d547" distance of L0.start L0.end
  measures "d548" distance of L2.end L0.start
  measures "d549" distance between parallel lines of L1 L4
  measures "d550" distance between parallel lines of L5 L6
  measures "d551" distance from line of L6 point (75, 60)
extrude "spectrometer lens stand" add sketch "Sketch166" along normal blind 79.74
sketch "Sketch167" plane through (105, 120, 0) normal (0, -1, 0) x (1, 0, 0)
  line L0 (0, 79.74) -> (20, 79.74) projected
  line L1 (2.5, 79.74) -> (2.5, 75.74)
  line L2 (2.5, 75.74) -> (17.5, 75.74)
  line L3 (17.5, 75.74) -> (17.5, 79.74)
  line L4 (17.5, 79.74) -> (2.5, 79.74)
  line L5 (0, 0) -> (0, 79.74) projected
  line L6 (20, 0) -> (20, 79.74) projected
  point P0 (-105, 0)
  dimension "d554" = 2.5
  dimension "d555" = 2.5
  dimension "d556" = 4
  constraints: 8 end point, 2 point on line, 1 perpendicular, 1 vertical
  measures "d554" distance between parallel lines of L5 L1
  measures "d555" distance between parallel lines of L6 L3
  measures "d556" distance between parallel lines of L0 L2
extrude "Extrusion111" cut sketch "Sketch167" against normal blind 20
sketch "Sketch168" plane through (107.5, 120, 75.74) normal (0, 0, 1) x (1, 0, 0)
  circle A0 centre (7.5, 10) radius 1.5
  line L0 (17.5, 0) -> (17.5, 20) projected
  line L1 (0, 20) -> (15, 20) projected
  point P0 (-107.5, -120)
  dimension "d559" = 10
  dimension "d560" = 10
  dimension "d561" = 3
  constraints: 1 centre point
  measures "d559" distance from line of A0.centre L0
  measures "d560" distance from line of L1 A0.centre
  measures "d561" diameter of A0
extrude "Extrusion112" cut sketch "Sketch168" against normal blind 50
thread "Thread8" size "5-40 UNC" class "2B" standard "ANSI Unified Screw Threads" full length
sketch "Sketch172" plane through (0, 0, 86.74) normal (0, 0, 1) x (1, 0, 0)
  line L0 (-30.5, 136) -> (-22.5, 136)
  line L1 (-22.5, 136) -> (-22.5, 124)
  line L2 (-22.5, 124) -> (-30.5, 124)
  line L3 (-30.5, 124) -> (-30.5, 136)
  line L4 (-20.5, 136) -> (-32.5, 136) projected
  line L5 (-32.5, 124) -> (-20.5, 124) projected
  line L6 (-32.5, 136) -> (-32.5, 124) projected
  line L7 (-20.5, 124) -> (-20.5, 136) projected
  point P0 (0, 0)
  dimension "d576" = 2
  dimension "d577" = 2
  constraints: 8 end point, 2 parallel, 2 point on line, 1 horizontal, 1 perpendicular
  measures "d576" distance between parallel lines of L6 L3
  measures "d577" distance between parallel lines of L7 L1
extrude "Extrusion113" cut sketch "Sketch172" against normal blind 4 contours L0 L1 L2 L3
sketch "Sketch173" plane through (0, 0, 150) normal (0, 0, 1) x (1, 0, 0)
  line L0 (0, -5) -> (0, 62) projected
  line L1 (42, 22) -> (42, 27) projected
  line L2 (0, 27) -> (42, 27)
  line L3 (42, 27) -> (42, 22)
  line L4 (42, 22) -> (0, 22)
  line L5 (0, 22) -> (0, 27)
  point P0 (0, 0)
  constraints: 8 end point, 2 parallel, 2 point on line, 1 horizontal, 1 perpendicular
extrude "Extrusion114" add sketch "Sketch173" against normal up to surface (150 mm away)
sketch "Sketch176" plane through (0, 0, 150) normal (0, 0, 1) x (1, 0, 0)
  line L0 (0, 65) -> (0, 27) projected
  line L1 (72, 27) -> (72, 65) projected
  line L2 (0, 45) -> (72, 45)
  line L3 (72, 45) -> (72, 55)
  line L4 (72, 55) -> (0, 55)
  line L5 (0, 55) -> (0, 45)
  line L6 (0, 65) -> (72, 65) projected
  point P0 (0, 0)
  point P1 (0, 55)
  dimension "d587" = 10
  dimension "d588" = 10
  constraints: 8 end point, 2 point on line, 1 horizontal, 1 parallel, 1 perpendicular
  measures "d587" distance between parallel lines of L4 L2
  measures "d588" distance between parallel lines of L4 L6
extrude "Extrusion116" add sketch "Sketch176" against normal up to surface (150 mm away) contours L4 L1 L2 L0
sketch "Sketch175" plane through (72, 0, 150) normal (0, 1, 0) x (1, 0, 0)
  line L0 (-50.9889, 37.496) -> (-0.9889, 37.496)
  line L1 (-0.9889, 37.496) -> (-0.9889, 87.496)
  line L2 (-0.9889, 87.496) -> (-50.9889, 87.496)
  line L3 (-50.9889, 87.496) -> (-50.9889, 37.496)
  point P0 (-72, 150)
  dimension "d582" = 50
  constraints: 8 end point, 2 parallel, 2 perpendicular, 1 horizontal
  measures "d582" distance of L2.end L0.start
extrude "Extrusion115" cut sketch "Sketch175" along normal blind 10 and the other way blind 10
sketch "Sketch179" plane through (0, 45, 150) normal (0, -1, 0) x (1, 0, 0)
  line L0 (71.0111, -37.496) -> (71.0111, -87.496) projected
  circle A0 centre (55, -50) radius 2.8 projected
  line L1 (12, -25) -> (62, -25)
  line L2 (62, -25) -> (62, -75)
  line L3 (62, -75) -> (12, -75)
  line L4 (12, -75) -> (12, -25)
  point P0 (0, -150)
  dimension "d593" = 16.0112
  dimension "d594" = 50
  dimension "d595" = 7
  dimension "d596" = 25
  constraints: 8 end point, 2 parallel, 2 perpendicular, 1 horizontal
  measures "d593" distance from line of L0 A0.centre
  measures "d594" distance of L3.end L1.start
  measures "d595" distance from line of L2 A0.centre
  measures "d596" distance from line of L1 A0.centre
extrude "Extrusion117" cut sketch "Sketch179" against normal blind 10 contours A0 | L1 L2 L3 L4
sketch "Sketch180" plane through (-35, 70, 150) normal (1, 0, 0) x (0, 0, -1)
  line L0 (66, 50) -> (66, 70) projected
  line L1 (66, 50) -> (69, 50)
  line L2 (69, 50) -> (69, 69.9941)
  line L3 (69, 69.9941) -> (66, 69.9941)
  line L4 (66, 69.9941) -> (66, 50)
  point P0 (150, -70)
  dimension "d599" = 3
  constraints: 8 end point, 2 parallel, 1 horizontal, 1 perpendicular
  measures "d599" distance of L2.end L3.end
extrude "Extrusion118" add sketch "Sketch180" against normal up to surface (25 mm away)
sketch "Sketch181" plane through (-35, 124, 88) normal (0, 0, 1) x (1, 0, 0)
  line L0 (-10.5, 0) -> (-22.5, 0)
  line L1 (-22.5, 0) -> (-22.5, 12)
  line L2 (-22.5, 12) -> (-10.5, 12)
  line L3 (-10.5, 12) -> (-10.5, 0)
  line L4 (0, 0) -> (-26, 0) projected
  line L5 (14.5, 0) -> (14.5, 12) projected
  line L6 (2.5, 12) -> (2.5, 0) projected
  point P0 (35, -124)
  dimension "d602" = 12
  dimension "d603" = 12
  dimension "d604" = 25
  constraints: 8 end point, 2 parallel, 2 perpendicular, 1 horizontal, 1 point on line
  measures "d602" distance of L0.end L1.end
  measures "d603" distance between parallel lines of L5 L6
  measures "d604" distance between parallel lines of L5 L3
extrude "Extrusion119" cut sketch "Sketch181" against normal blind 3